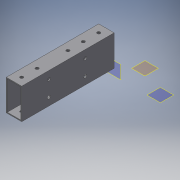
# Autodesk Inventor part: left arm
Saved by Autodesk Inventor 2018 (Build 220112000, 112)
## iProperties
Created: 2019-01-16
Part Number: left arm
Material: Generic
Document SubType Name: Modeling
Designer: s-4008082
Density: 1 g/cm^3
Appearance: Default
Mass: 126.635 g
Surface Area: 952.38 cm^2
Volume: 126.635 cm^3
Author: s-4008082
Autodesk Inventor part; units mm, degrees
ref_plane "YZ Plane" through (0, 0, 0) normal (1, 0, 0) x (0, 1, 0)
ref_plane "XZ Plane" through (0, 0, 0) normal (0, 1, 0) x (-1, 0, 0)
ref_plane "XY Plane" through (0, 0, 0) normal (0, 0, 1) x (1, 0, 0)
ref_plane "Work Plane1" through (0, 0, 0) normal (0, 0, -1) x (-1, 0, 0)
sketch "Sketch20" plane through (0, 0, 0) normal (0, 0, -1) x (-1, 0, 0)
  line L0 (0, 0) -> (25.4, 0)
  line L1 (25.4, 0) -> (0, 0)
  line L2 (0, 0) -> (0, 50.8)
  line L3 (0, 50.8) -> (25.4, 50.8)
  line L4 (25.4, 50.8) -> (25.4, 0)
  line L5 (23.749, 49.149) -> (1.651, 49.149)
  line L6 (1.651, 49.149) -> (1.651, 1.651)
  line L7 (1.651, 1.651) -> (23.749, 1.651)
  line L8 (23.749, 1.651) -> (23.749, 49.149)
  line L9 (0, 0) -> (0, 50.8) projected
  dimension "d71" = 25.4
  dimension "d72" = 50.8
  dimension "d73" = 1.651
  dimension "d74" = 1.651
  dimension "d75" = 1.651
  dimension "d76" = 1.651
  dimension "d78" = 0
  constraints: 18 end point, 4 parallel, 2 horizontal, 2 perpendicular
  measures "d71" distance of L2.end L3.end
  measures "d72" distance of L1.end L2.end
  measures "d73" distance between parallel lines of L3 L5
  measures "d74" distance between parallel lines of L2 L6
  measures "d75" distance between parallel lines of L1 L7
  measures "d76" distance between parallel lines of L4 L8
  measures "d78" distance between parallel lines of L9 L2
extrude "Extrusion16" add sketch "Sketch20" against normal blind 152.4
ref_plane "Work Plane4" through (76.2, 0, 0) normal (0, -1, 0) x (1, 0, 0)
sketch "Sketch21" plane through (76.2, 0, 0) normal (0, -1, 0) x (1, 0, 0)
  circle A0 centre (-38.1, 12.7) radius 2.5797
  circle A1 centre (-63.5, 12.7) radius 2.5797
  circle A2 centre (-88.9, 12.7) radius 2.5797
  circle A3 centre (-88.9, 38.1) radius 2.5797
  circle A4 centre (-88.9, 63.5) radius 2.5797
  line L0 (-76.2, 25.4) -> (0, 25.4) projected
  line L1 (-101.6, 0) -> (-101.6, 152.4) projected
  line L2 (-76.2, 25.4) -> (-76.2, 152.4) projected
  point P0 (-76.2, 0)
  dimension "d81" = 12.7
  dimension "d82" = 12.7
  dimension "d83" = 12.7
  dimension "d84" = 25.4
  dimension "d85" = 12.7
  dimension "d86" = 5.1594
  dimension "d87" = 5.1594
  dimension "d88" = 5.1594
  dimension "d89" = 25.4
  dimension "d90" = 25.4
  dimension "d91" = 25.4
  dimension "d92" = 5.1594
  dimension "d93" = 5.1594
  dimension "d94" = 12.7
  dimension "d95" = 12.7
  constraints: 5 centre point
  measures "d81" distance from line of L0 A0.centre
  measures "d82" distance from line of L0 A2.centre
  measures "d83" distance from line of L1 A2.centre
  measures "d84" distance of A2.centre A1.centre
  measures "d85" distance from line of L0 A1.centre
  measures "d86" diameter of A0
  measures "d87" diameter of A1
  measures "d88" diameter of A2
  measures "d89" distance of A1.centre A0.centre
  measures "d90" distance of A2.centre A3.centre
  measures "d91" distance of A3.centre A4.centre
  measures "d92" diameter of A4
  measures "d93" diameter of A3
  measures "d94" distance from line of L2 A3.centre
  measures "d95" distance from line of L2 A4.centre
extrude "Extrusion17" cut sketch "Sketch21" against normal blind 76.2
ref_plane "Work Plane3" through (-25.4, 0, 0) normal (-1, 0, 0) x (0, 0, 1)
sketch "Sketch26" plane through (-25.4, 0, 0) normal (-1, 0, 0) x (0, 0, 1)
  circle A0 centre (107.569, 38.1) radius 2.5797
  line L0 (152.4, 50.8) -> (152.4, 0) projected
  line L1 (0, 50.8) -> (152.4, 50.8) projected
  circle A1 centre (47.752, 38.1) radius 2.5797
  circle A2 centre (107.569, 12.7) radius 2.5797
  circle A3 centre (47.752, 12.7) radius 2.5797
  point P0 (0, 0)
  dimension "d122" = 5.1594
  dimension "d123" = 44.831
  dimension "d124" = 12.7
  dimension "d125" = 5.1594
  dimension "d126" = 59.817
  dimension "d129" = 25.4
  dimension "d130" = 5.1594
  dimension "d131" = 25.4
  dimension "d132" = 5.1594
  dimension "d143" = 12.7
  constraints: 4 centre point
  measures "d122" diameter of A0
  measures "d123" distance from line of L0 A0.centre
  measures "d124" distance from line of L1 A0.centre
  measures "d125" diameter of A1
  measures "d126" distance of A0.centre A1.centre
  measures "d129" distance of A0.centre A2.centre
  measures "d130" diameter of A2
  measures "d131" distance of A1.centre A3.centre
  measures "d132" diameter of A3
  measures "d143" distance from line of L1 A1.centre
extrude "Extrusion22" cut sketch "Sketch26" against normal blind 25.4
ref_plane "Work Plane2" through (76.2, 50.8, 25.4) normal (0, 1, 0) x (1, 0, 0)
sketch "Sketch27" plane through (76.2, 50.8, 25.4) normal (0, 1, 0) x (1, 0, 0)
  circle A0 centre (-88.9, -114.3) radius 2.5797
  circle A1 centre (-88.9, -88.9) radius 2.5797
  line L0 (-76.2, -127) -> (-101.6, -127) projected
  line L1 (-76.2, 0) -> (-76.2, -127) projected
  point P0 (-76.2, 25.4)
  dimension "d135" = 12.7
  dimension "d136" = 12.7
  dimension "d137" = 38.1
  dimension "d138" = 12.7
  dimension "d139" = 5.1594
  dimension "d140" = 5.1594
  constraints: 2 centre point
  measures "d135" distance from line of L0 A0.centre
  measures "d136" distance from line of L1 A0.centre
  measures "d137" distance from line of L0 A1.centre
  measures "d138" distance from line of L1 A1.centre
  measures "d139" diameter of A1
  measures "d140" diameter of A0
extrude "Extrusion23" cut sketch "Sketch27" against normal blind 50.8
equation "\"d74\" = d73"
equation "\"d75\" = d73"
equation "\"d76\" = d73"
equation "\"d87\" = d86"
equation "\"d88\" = d86"
equation "\"d92\" = d86"
equation "\"d93\" = d86"
equation "\"d125\" = d122"
equation "\"d130\" = d122"
equation "\"d132\" = d122"
equation "\"d140\" = d139"
body "Solid2"
